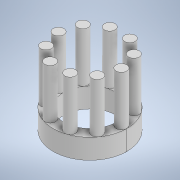
# Autodesk Inventor part: piece_roue_test_2
Saved by Autodesk Inventor 2020.1 (Build 241239000, 239)
## iProperties
Created: 2019-07-25
Part Number: piece_roue_test_2
Material: Générique
Document SubType Name: Modeling
Designer: marlo
Density: 1 g/cm^3
Appearance: Par défaut
Author: marlo
Autodesk Inventor part; units mm, degrees
ref_plane "YZ Plane" through (0, 0, 0) normal (1, 0, 0) x (0, 1, 0)
ref_plane "XZ Plane" through (0, 0, 0) normal (0, 1, 0) x (-1, 0, 0)
ref_plane "XY Plane" through (0, 0, 0) normal (0, 0, 1) x (1, 0, 0)
sketch "Esquisse1" plane through (0, 0, 0) normal (0, 1, 0) x (-1, 0, 0)
  circle A0 centre (0, 0) radius 2.7
  dimension "d0" = 5.4
  constraints: 1 centre point, 1 coincident
  measures "d0" diameter of A0
extrude "Extrusion1" add sketch "Esquisse1" along normal blind 25
sketch "Esquisse2" plane through (0, 0, 0) normal (0, -1, 0) x (1, 0, 0)
  line L0 (2.7, 5.0753) -> (2.7, -12.6206) construction
  circle A0 centre (0, 0) radius 2.7 projected
  circle A1 centre (-15.8, 0) radius 18.5
  line L1 (8.7278, 0) -> (-17.8614, 0) construction
  point P0 (2.7, 0)
  dimension "d4" = 37
  constraints: 4 end point, 2 point on line, 2 tangent, 1 centre point, 1 horizontal, 1 vertical
  measures "d4" diameter of A1
extrude "Extrusion2" add sketch "Esquisse2" along normal blind 10
sketch "Esquisse3" plane through (-15.8, 0, 0) normal (0, 1, 0) x (1, 0, 0)
  line L0 (-18.5, -20.7984) -> (-18.5, 1.736) construction
  circle A0 centre (-12.8328, 9.2173) radius 2.7
  circle A1 centre (-15.8, 0) radius 2.7
  circle A2 centre (-5.0457, 14.9727) radius 2.7
  line L1 (-5.0457, 14.9727) -> (-12.8328, 9.2173) construction
  line L2 (-12.8328, 9.2173) -> (-15.8, 0) construction
  line L3 (-15.8, 0) -> (0, 0) construction
  line L4 (-12.8328, 9.2173) -> (0, 0) construction
  line L5 (-5.0457, 14.9727) -> (0, 0) construction
  line L6 (-15.8, 0) -> (-18.5, 0) construction
  line L7 (-12.8328, 9.2173) -> (-15.0195, 10.8011) construction
  line L8 (-5.0457, 14.9727) -> (-7.4489, 16.2034) construction
  line L9 (0, 30.0966) -> (0, -33.1039)
  line L10 (-38.9474, 0) -> (38.9474, 0)
  circle A3 centre (12.8328, 9.2173) radius 2.7
  circle A4 centre (5.0457, 14.9727) radius 2.7
  circle A5 centre (-12.8328, -9.2173) radius 2.7
  circle A6 centre (-5.0457, -14.9727) radius 2.7
  circle A7 centre (5.0457, -14.9727) radius 2.7
  circle A8 centre (12.8328, -9.2173) radius 2.7
  circle A9 centre (0, 0) radius 18.5 projected
  point P0 (18.5, 0)
  dimension "d14" = 5.4
  constraints: 22 end point, 6 centre point, 6 symmetric about line, 5 equal length, 4 vertical, 2 horizontal, 2 horizontal alignment, 1 coincident, 1 midpoint, 14 other
extrude "Extrusion3" add sketch "Esquisse3" along normal blind 25 contours A0 | A2 | L10 A1 | A1 L10 | A5 | A6 | A3 | A4 | A7 | A8
sketch "Esquisse4" plane through (-15.8, -10, 0) normal (0, -1, 0) x (1, 0, 0)
  circle A0 centre (15.8, 0) radius 2.65
  constraints: 1 centre point, 1 coincident
extrude "Extrusion4" add sketch "Esquisse4" against normal blind 10
sketch "Esquisse5" plane through (0, 0, 0) normal (0, 1, 0) x (1, 0, 0)
  circle A0 centre (-15.8, 0) radius 13.1
  arc A1 (-9.892, 17.5313) -> (-21.708, 17.5313) centre (-15.8, 0) ccw projected
  circle A2 centre (-2.9672, 9.2173) radius 2.7 projected
  point P0 (0, 0)
  constraints: 1 centre point, 1 concentric, 1 tangent
extrude "Extrusion5" cut sketch "Esquisse5" against normal blind 10 contours A0
